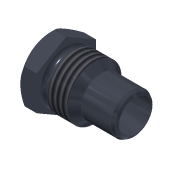
# Autodesk Inventor part: Cap03
Saved by Autodesk Inventor 2019 (Build 230136000, 136)
## iProperties
Company: RIVETEC s.r.o.
Category: Naradi
Created: 2007-11-20
Part Number: Cap03
Cost Center: 0,006 kg
Material: ČSN 12 050 (1.1201, C45)
Document SubType Name: Modeling
Designer: matousek
Mass: 7.12897 g
Surface Area: 8.98233 cm^2
Volume: 0.909307 cm^3
Density: 7.84 g/cm^3
Description: náustek 6,4
Stock Number: 10-0252
Appearance: Černěno
Vendor: RIVETEC s.r.o.
Hrubá hmotnost: 0,016 kg
VV: 00
ZměnovéŘízení: -
NázevAnglicky: MOUTH
Datum uložení: 2007-11-19
Čas uložení: 11:47
Jméno souboru: 10-0252_0171031000
Hmotnost: 0,006 kg
LastSaveDate: 2016-11-23
Mass: 0
FileName: 10-0252_0171031000
Tep_zprac: KALIT, POPUSTIT 45 HRC
Povrch_U: ČERNIT
Tolerance: ISO 2768-mK
Author: matousek
Last Saved By: navara
Autodesk Inventor part; units mm, degrees
ref_plane "YZ Plane" through (0, 0, 0) normal (1, 0, 0) x (0, 1, 0)
ref_plane "XZ Plane" through (0, 0, 0) normal (0, 1, 0) x (-1, 0, 0)
ref_plane "XY Plane" through (0, 0, 0) normal (0, 0, 1) x (1, 0, 0)
sketch "Náčrt1" plane through (0, 0, 0) normal (0, 0, 1) x (1, 0, 0)
  line L0 (0, 0) -> (0, 2.5)
  line L1 (0, 2.5) -> (0.555, 3.4613)
  line L2 (6.6, 3.75) -> (7.85, 5)
  line L3 (7.85, 5) -> (11.6, 5)
  line L4 (11.6, 5) -> (11.6, 4.95)
  arc A0 (11.6, 4.95) -> (13.1, 4.95) centre (12.35, 4.95) ccw
  line L5 (13.1, 4.95) -> (13.1, 6.5)
  line L6 (13.1, 6.5) -> (17.1, 6.5)
  line L7 (17.1, 6.5) -> (17.1, 0)
  line L8 (17.1, 0) -> (0, 0)
  line L9 (1.055, 3.75) -> (0.555, 3.4613)
  line L10 (1.055, 3.75) -> (6.6, 3.75)
  arc A1 (17.1, 2.5) -> (15.1, 6.5) centre (12.1, 2.5) ccw
  dimension "d2" = 30
  dimension "d3" = 45
  dimension "d5" = 6.6
  dimension "d6" = 10
  dimension "d7" = 5
  dimension "d8" = 1.5
  dimension "d9" = 13.1
  dimension "d10" = 17.1
  dimension "d11" = 13
  dimension "d12" = 8.4
  dimension "d32" = 30
  dimension "d34" = 0.5
  dimension "d35" = 7.5
  dimension "d46" = 5
  dimension "d47" = 5
  constraints: 22 end point, 6 parallel, 4 point on circle, 3 tangent, 2 centre point, 1 midpoint, 1 perpendicular, 1 point on line, 1 vertical
  measures "d2" angle of L0 L1
  measures "d3" angle of L3 L2
  measures "d5" distance from line of L2.start L0
  measures "d6" diameter of L3 L8
  measures "d7" diameter of L0.end L8
  measures "d8" distance between parallel lines of L5 L4
  measures "d9" distance between parallel lines of L5 L0
  measures "d10" distance between parallel lines of L7 L0
  measures "d11" diameter of L6 L8
  measures "d32" angle of L8 L9
  measures "d34" horizontal distance of L9.start L1.end
  measures "d35" diameter of L10 L8
  measures "d46" radius of A1
  measures "d47" diameter of A1.start L8
revolve "Rotace1" add sketch "Náčrt1" angle 360 about axis through (17.1, 0, 0) along (-1, 0, 0) contours L0 L1 L9 L10 L2 L3 L4 A0 L5 L6 A1 L7 L8
sketch "Náčrt2" plane through (17.1, 0, 0) normal (1, 0, 0) x (0, 0, -1)
  line L0 (3.1754, 5.5) -> (6.3509, 0)
  line L1 (6.3509, 0) -> (3.1754, -5.5)
  line L2 (3.1754, -5.5) -> (-3.1754, -5.5)
  line L3 (-3.1754, -5.5) -> (-6.3509, 0)
  line L4 (-6.3509, 0) -> (-3.1754, 5.5)
  line L5 (-3.1754, 5.5) -> (3.1754, 5.5)
  circle A0 centre (0, 0) radius 7.7861
  dimension "d14" = 5.5
  constraints: 12 end point, 2 coincident, 1 centre point, 13 other
  measures "d14" distance from line of L5 point (0, 0)
extrude "Vysunutí1" cut sketch "Náčrt2" against normal through all
sketch "Náčrt4" plane through (0, 0, 0) normal (-1, 0, 0) x (0, 0, 1)
  circle A0 centre (0, 0) radius 3.75 projected
  point P0 (0, 0)
  constraints: 1 coincident
hole "Díra1" at (0, 0, 0) direction (1, 0, 0) diameter 6 end through all
thread "Závit1" size "M10x1" class "6g" standard "ISO Metric profile" full length
move or copy body "Posunout těleso1" bodies to move or copy 1 copy no rotation origin (0, 0, 0) rotation axis (0, 0, 1) rotation angle 180 translate (13.1, 0, 0)
